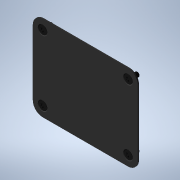
# Autodesk Inventor part: SCHUNK-5524251 Abdeckblech-PGN-plus-P 160
Saved by Autodesk Inventor 2021 (Build 250183000, 183)
## iProperties
Created: 2025-07-30
Part Number: SCHUNK-5524251 Abdeckblech-PGN-plus-P 160
Material: Generic
Catalog Web Link: www.cadenas.de
Description: Abdeckblech PGN-plus P-2-finger parallel gripper
Vendor: SCHUNK
Document SubType Name: Modeling
Designer: psAdmin
Manufacturer: SCHUNK
Mass: 3.17929 g
Surface Area: 80.4427 cm^2
Volume: 3.17929 cm^3
Density: 1 g/cm^3
Appearance: PSOLRGB-175-175-175
Category: PARTsolutions
Company: SCHUNK
Title: SCHUNK-5524251 Abdeckblech-PGN-plus-P 160
Author: Cadenas PARTsolutions
Comments: 2-finger parallel gripper
PSOL_IDENT_0: {$CADENAS_DATA/23d-libs/schunk/greifsysteme/greifmodule/greifmodule_pneumatisch/2_finger_parallelgre
PSOL_IDENT_1: ifer/2_finger_universalgreifer/pgn_plus_p/pgnplus_p_adb.prj},238 {VTYP=3D},{NB=SCHUNK-5524251 Abdeck
PSOL_IDENT_2: blech-PGN-plus-P 160},{LINA=SCHUNK-5524251 Abdeckblech-PGN-plus-P 160},{NN=Abdeckblech PGN-plus P},{
PSOL_IDENT_3: DATE=24.02.2025 16:11:11},{GEOMDATE=17.05.2022 13:48:12},{VERSION=},{LINEID=80},{WBVAR=},{WBNUMERIC=
PSOL_IDENT_4: }  {NB=SCHUNK-5524251 Abdeckblech-PGN-plus-P 160},{LINA=SCHUNK-5524251 Abdeckblech-PGN-plus-P 160},{
PSOL_IDENT_5: KT=DUMMY},{IDNR=5524251},{TYP=PGN-plus-P 160},{L=68.800},{B=55.800},{H=0.800},{R1=6.400},{LS1=28.000
PSOL_IDENT_6: },{LS2=21.500},{SD1=6.300},{LS3=0.150},{DSK=5.500},{HSK=1.650},{GS=3.000},{LS=6.000},{TKT=1.500},{D1=
PSOL_IDENT_7: 0.900},{D2=0.600},{TT=0.800},{TYP1=8.000},{CNSCTN=84799020}
NB: SCHUNK-5524251 Abdeckblech-PGN-plus-P 160
NN: Abdeckblech PGN-plus P
NT: 2-finger parallel gripper
NBSYN: SCHUNK-$IDNR. Abdeckblech-$TYP.
LINA: SCHUNK-5524251 Abdeckblech-PGN-plus-P 160
CATALOG: SCHUNK
IDNR: 5524251
TYP: PGN-plus-P 160
L: 68.8
B: 55.8
H: 0.8
R1: 6.4
LS1: 28
LS2: 21.5
SD1: 6.3
LS3: 0.15
DSK: 5.5
HSK: 1.65
GS: 3
LS: 6
TKT: 1.5
D1: 0.9
D2: 0.6
TT: 0.8
TYP1: 8
CNSCTN: 84799020
SUPPLIER: SCHUNK
ARTICLENO: SCHUNK-5524251 Abdeckblech-PGN-plus-P 160
BOMINFO: SCHUNK-5524251 Abdeckblech-PGN-plus-P 160
CREATOR: CADENAS GmbH
Autodesk Inventor part; units mm, degrees
sketch "Sketch_1" plane through (0, 0, 0) normal (0, 0, 1) x (1, 0, 0)
  line L0 (-34.4, 21.5) -> (-34.4, -21.5)
  arc A0 (-34.4, -21.5) -> (-28, -27.9) centre (-28, -21.5) ccw
  line L1 (-28, -27.9) -> (28, -27.9)
  arc A1 (28, -27.9) -> (34.4, -21.5) centre (28, -21.5) ccw
  line L2 (34.4, -21.5) -> (34.4, 21.5)
  arc A2 (34.4, 21.5) -> (28, 27.9) centre (28, 21.5) ccw
  line L3 (28, 27.9) -> (-28, 27.9)
  arc A3 (-28, 27.9) -> (-34.4, 21.5) centre (-28, 21.5) ccw
  constraints: 8 end point, 8 point on circle, 4 centre point
extrude "Extrusion1" add sketch "Sketch_1" along normal blind 0.8
sketch "Sketch_2" plane through (28, 0, 0) normal (1, 0, 0) x (0, 0, -1)
  line L0 (0, 21.5) -> (-0.8, 21.5)
  line L1 (-0.8, 21.5) -> (-0.8, 24.65)
  line L2 (-0.8, 24.65) -> (0, 23.85)
  line L3 (0, 23.85) -> (0, 21.5)
  line L4 (0, 21.5) -> (-0.8, 21.5)
  constraints: 10 end point
revolve "Revolution1" cut sketch "Sketch_2" angle 360 about axis through (28, 21.5, 0) along (0, 0, -1)
pattern_linear "Rectangular Pattern1" count 2 spacing 56 along (-1, 0, 0) count 2 spacing 43 along (0, -1, 0) of "Revolution1"
sketch "Sketch_4" plane through (28, 0, 0) normal (1, 0, 0) x (0, 0, -1)
  line L0 (5.35, 21.5) -> (-0.65, 21.5)
  line L1 (-0.65, 21.5) -> (-0.65, 24.25)
  line L2 (-0.65, 24.25) -> (-0.25, 24.25)
  line L3 (-0.25, 24.25) -> (1, 23)
  line L4 (1, 23) -> (5.15, 23)
  line L5 (5.15, 23) -> (5.35, 22.8)
  line L6 (5.35, 22.8) -> (5.35, 21.5)
  line L7 (5.35, 21.5) -> (-0.65, 21.5)
  constraints: 16 end point
revolve "Revolution2" add sketch "Sketch_4" angle 360 about axis through (28, 21.5, -5.35) along (0, 0, -1)
thread "Thread1" size "M3x0.5" class "6g" standard "ISO Metric profile" full length
pattern_linear "Rectangular Pattern2" count 2 spacing 56 along (-1, 0, 0) count 2 spacing 43 along (0, -1, 0) of "Revolution2"
sketch "Sketch_6" plane through (0, 0, 0.65) normal (0, 0, 1) x (1, 0, 0)
  arc A0 (27.025, 22.4093) -> (26.725, 21.8897) centre (26.875, 22.1495) ccw
  arc A1 (26.725, 21.1103) -> (26.725, 21.8897) centre (26.5, 21.5) ccw
  arc A2 (26.725, 21.1103) -> (27.025, 20.5907) centre (26.875, 20.8505) ccw
  arc A3 (27.7, 20.201) -> (27.025, 20.5907) centre (27.25, 20.201) ccw
  arc A4 (27.7, 20.201) -> (28.3, 20.201) centre (28, 20.201) ccw
  arc A5 (28.975, 20.5907) -> (28.3, 20.201) centre (28.75, 20.201) ccw
  arc A6 (28.975, 20.5907) -> (29.275, 21.1103) centre (29.125, 20.8505) ccw
  arc A7 (29.275, 21.8897) -> (29.275, 21.1103) centre (29.5, 21.5) ccw
  arc A8 (29.275, 21.8897) -> (28.975, 22.4093) centre (29.125, 22.1495) ccw
  arc A9 (28.3, 22.799) -> (28.975, 22.4093) centre (28.75, 22.799) ccw
  arc A10 (28.3, 22.799) -> (27.7, 22.799) centre (28, 22.799) ccw
  arc A11 (27.025, 22.4093) -> (27.7, 22.799) centre (27.25, 22.799) ccw
  constraints: 24 point on circle, 12 centre point
extrude "Extrusion2" cut sketch "Sketch_6" against normal blind 0.8
pattern_linear "Rectangular Pattern3" count 2 spacing 56 along (-1, 0, 0) count 2 spacing 43 along (0, -1, 0) of "Extrusion2"
ref_plane "einbau_XY" through (0, 0, 0) normal (0, 0, 1) x (1, 0, 0)
ref_plane "einbau_YZ" through (0, 0, 0) normal (1, 0, 0) x (0, 1, 0)
ref_plane "einbau_ZX" through (0, 0, 0) normal (0, 1, 0) x (0, 0, 1)
body "Solid1"
